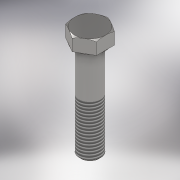
# Autodesk Inventor part: SCREW M24x120-01-02
Saved by Autodesk Inventor 2022.2 (Build 262287010, 287A)
## iProperties
Created: 2022-12-19
Part Number: SCREW M24x120-01-02
Material: Steel
Document SubType Name: Modeling
Designer: User
Mass: 527.789 g
Surface Area: 152.44 cm^2
Volume: 67.2343 cm^3
Density: 7.85 g/cm^3
Appearance: Semi-Polished
Author: User
Autodesk Inventor part; units mm, degrees
ref_plane "YZ Plane" through (0, 0, 0) normal (1, 0, 0) x (0, 1, 0)
ref_plane "XZ Plane" through (0, 0, 0) normal (0, 1, 0) x (-1, 0, 0)
ref_plane "XY Plane" through (0, 0, 0) normal (0, 0, 1) x (1, 0, 0)
sketch "Sketch1" plane through (0, 0, 0) normal (0, 1, 0) x (-1, 0, 0)
  line L0 (127.8939, 73.8396) -> (127.8939, -73.8396)
  line L1 (127.8939, -73.8396) -> (0, -147.6791)
  line L2 (0, -147.6791) -> (-127.8939, -73.8396)
  line L3 (-127.8939, -73.8396) -> (-127.8939, 73.8396)
  line L4 (-127.8939, 73.8396) -> (0, 147.6791)
  line L5 (0, 147.6791) -> (127.8939, 73.8396)
  line L6 (-16, 9.2376) -> (0, 18.4752)
  line L7 (0, 18.4752) -> (16, 9.2376)
  line L8 (16, 9.2376) -> (16, -9.2376)
  line L9 (16, -9.2376) -> (0, -18.4752)
  line L10 (0, -18.4752) -> (-16, -9.2376)
  line L11 (-16, -9.2376) -> (-16, 9.2376)
  point P0 (0, 0)
  point P1 (0, 0)
  point P2 (0, 0)
  dimension "Shex" = 32
  constraints: 24 end point, 2 coincident, 2 vertical, 26 other
  measures "Shex" distance between parallel lines of L11 L8
extrude "Extrusion1" add sketch "Sketch1" along normal blind 14 contours L6 L7 L8 L9 L10 L11
sketch "Sketch2" plane through (0, 0, 0) normal (1, 0, 0) x (0, 1, 0)
  line L0 (0, -18.4752) -> (14, -18.4752) construction
  line L1 (14, -18.4752) -> (12.5709, -18.4752)
  line L2 (12.5709, -18.4752) -> (14, -16)
  line L3 (14, -16) -> (14, -18.4752)
  line L4 (-3, 0) -> (18, 0) projected
  point P0 (0, 0)
  dimension "d4" = 60
  dimension "d5" = 32
  constraints: 6 end point, 1 point on line, 1 vertical
  measures "d4" angle of L2 L0
  measures "d5" diameter of L2.end L4
revolve "Revolution1" cut sketch "Sketch2" angle 360 about axis through (0, -10, 0) along (0, 1, 0)
sketch "Sketch3" plane through (0, 0, 0) normal (0, 0, 1) x (1, 0, 0)
  line L0 (0, 0) -> (11, 0)
  line L1 (11, 0) -> (11, -100)
  line L2 (11, -100) -> (0, -100)
  line L3 (0, -100) -> (0, 0)
  dimension "L" = 100
  dimension "Dia" = 22
  constraints: 8 end point, 2 parallel, 1 horizontal, 1 perpendicular
  measures "L" distance of L0.end L1.end
  measures "Dia" diameter of L1 L3
revolve "Revolution2" add sketch "Sketch3" angle 360 about axis through (0, -100, 0) along (0, 1, 0)
fillet "Fillet1" radius 0.7 1 edges at (-11, 0, 0)
chamfer "Chamfer1" distance 2 angle 45 1 edges at (-11, -100, 0)
thread "Thread2" size "M24x3" class "6g" standard "ANSI Metric M Profile" length 52
sketch "Sketch6" plane through (0, 0, 0) normal (1, 0, 0) x (0, 1, 0)
  line L0 (-3.0757, 0) -> (18.4544, 0) projected
  line L1 (0, -18.4752) -> (12.5709, -18.4752) projected
  line L2 (0, -18.4752) -> (0, -9.2376) projected
  line L3 (0, -9.2376) -> (12.5709, -9.2376) projected
  line L4 (0, -18.4752) -> (0.5, -18.4752)
  line L5 (0.5, -18.4752) -> (0.5, -16)
  line L6 (0.5, -16) -> (0, -16)
  line L7 (0, -16) -> (0, -18.4752)
  point P0 (0, 0)
  point P1 (14, -13.8564)
  point P2 (0, -16)
  dimension "a" = 0.5
  dimension "d34" = 32
  constraints: 8 end point, 2 parallel, 1 horizontal, 1 perpendicular, 2 other
  measures "a" distance of L6.end L5.end
  measures "d34" diameter of L6 L0
revolve "Revolution3" cut sketch "Sketch6" angle 360 about axis through (0, -10, 0) along (0, 1, 0)
equation "\"d5\" = Shex"
equation "\"d31\" = b - cham"
equation "\"d34\" = Shex"
equation "\"b\" = 54"
equation "\"cham\" = 2"
body "Solid1"
